# Autodesk Inventor part: RF4463F30
Saved by Autodesk Inventor 2015 SP1 (Build 190203100, 203)
## iProperties
Created: 2015-10-19
Part Number: RF4463F30
Material: Generic
Document SubType Name: Modeling
Designer: Kartikye
Density: 1 g/cm^3
Appearance: RF4463F30, RF4463F30
Author: Kartikye
Autodesk Inventor part; units mm, degrees
ref_plane "YZ Plane" through (0, 0, 0) normal (1, 0, 0) x (0, 1, 0)
ref_plane "XZ Plane" through (0, 0, 0) normal (0, 1, 0) x (-1, 0, 0)
ref_plane "XY Plane" through (0, 0, 0) normal (0, 0, 1) x (1, 0, 0)
sketch "RF4463F30, RF4463F30_7" plane through (0, 0, 0) normal (0, 0, 1) x (1, 0, 0)
  line L0 (-0.25, 0.25) -> (38, 0.25)
  line L1 (38, 0.25) -> (38, -26.9142)
  line L2 (38, -26.9142) -> (-0.25, -26.9142)
  line L3 (-0.25, -26.9142) -> (-0.25, 0.25)
  constraints: 8 end point
extrude "Extrusion1" add sketch "RF4463F30, RF4463F30_7" along normal blind 1
body "Solid1"
